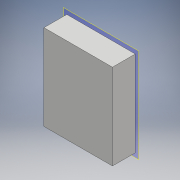
# Autodesk Inventor part: BaseCuello
Saved by Autodesk Inventor 2017 SP1 (Build 210196100, 196)
## iProperties
Part Number: BaseCuello
Material: Genérico
Document SubType Name: Modeling
Designer: Juan
Density: 1 g/cm^3
Appearance: Valor por defecto
Author: Juan
Autodesk Inventor part; units mm, degrees
ref_plane "YZ Plane" through (0, 0, 0) normal (1, 0, 0) x (0, 1, 0)
ref_plane "XZ Plane" through (0, 0, 0) normal (0, 1, 0) x (-1, 0, 0)
ref_plane "XY Plane" through (0, 0, 0) normal (0, 0, 1) x (1, 0, 0)
sketch "Boceto1" plane through (0, 0, 0) normal (0, 1, 0) x (-1, 0, 0)
  line L0 (120, 150) -> (0, 150)
  line L1 (0, 150) -> (0, 0)
  line L2 (0, 0) -> (120, 0)
  line L3 (120, 0) -> (120, 150)
  dimension "d0" = 120
  dimension "d1" = 150
  constraints: 8 end point, 2 parallel, 1 coincident, 1 horizontal, 1 perpendicular
  measures "d0" distance of L2.end L1.end
  measures "d1" distance of L0.end L1.end
extrude "Extrusión1" add sketch "Boceto1" along normal blind 40
ref_plane "Plano de trabajo1" through (0, 40, 0) normal (0, 1, 0) x (1, 0, 0)
sketch "Boceto2" plane through (0, 40, 0) normal (0, 1, 0) x (1, 0, 0)
  line L0 (-120, -150) -> (-80, -150) construction
  line L1 (0, -150) -> (-40, -150) construction
  line L2 (-80, -150) -> (-80, -144.987) construction
  line L3 (-40, -150) -> (-40, -144.987) construction
  line L4 (-80, -144.987) -> (-40, -144.987)
  line L5 (-40, -144.987) -> (-40, -124.987)
  line L6 (-40, -124.987) -> (-80, -124.987)
  line L7 (-80, -124.987) -> (-80, -144.987)
  point P0 (0, 0)
  dimension "d6" = 40
  dimension "d8" = 20
  constraints: 16 end point, 3 perpendicular, 2 vertical, 1 horizontal
  measures "d6" distance of L1.start L1.end
  measures "d8" distance of L3.end L5.end
extrude "Extrusión2" cut sketch "Boceto2" against normal blind 27
ref_plane "Plano de trabajo2" through (-80, 13, 144.987) normal (1, 0, 0) x (0, 0, -1)
sketch "Boceto3" plane through (-80, 13, 144.987) normal (1, 0, 0) x (0, 0, -1)
  line L0 (0, 27) -> (0, 7) construction
  line L1 (0, 27) -> (0, 0) construction
  line L2 (0, 7) -> (13, 7) construction
  line L3 (20, 27) -> (20, 0) construction
  line L4 (20, 27) -> (20, 7) construction
  line L5 (20, 7) -> (7, 7) construction
  line L6 (7, 7) -> (13, 7)
  line L7 (13, 7) -> (13, 3)
  line L8 (13, 3) -> (7, 3)
  line L9 (7, 3) -> (7, 7)
  point P0 (144.987, -13)
  dimension "d12" = 20
  dimension "d13" = 13
  dimension "d14" = 20
  dimension "d15" = 13
  dimension "d16" = 4
  constraints: 16 end point, 2 perpendicular, 2 point on line, 1 collinear, 1 horizontal, 1 vertical
  measures "d12" distance of L0.start L0.end
  measures "d13" distance of L0.end L2.end
  measures "d14" distance of L3.start L4.end
  measures "d15" distance of L4.end L5.end
  measures "d16" distance of L2.end L7.end
extrude "Extrusión3" cut sketch "Boceto3" against normal blind 45
sketch "Boceto4" plane through (0, 40, 0) normal (0, 1, 0) x (1, 0, 0)
  line L0 (0, 0) -> (-120, 0) projected
  line L1 (-60, 0) -> (-60, -60) construction
  circle A0 centre (-60, -60) radius 51
  dimension "d20" = 60
  dimension "d21" = 102
  constraints: 2 end point, 1 centre point, 1 coincident, 1 midpoint, 1 vertical
  measures "d20" distance of L1.start L1.end
  measures "d21" diameter of A0
extrude "Extrusión4" cut sketch "Boceto4" against normal blind 30
